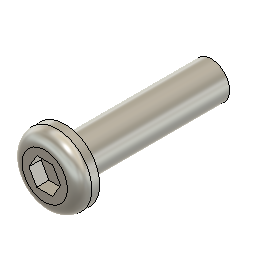
_bolt.35465e34-b387-4346-8fbb-dc58b0572cbc (Autodesk Fusion 360 design; units mm, degrees)
Autodesk Fusion 360 part; units mm, degrees
sketch "Sketch1" plane through (0, 0, 0) normal (0, 0, 1) x (1, 0, 0)
  circle A0 centre (0, 0) radius 2.85
  dimension "d1" = 5.7
  constraint coincident A0.centre origin
  measures "d1" diameter of A0
extrude "Extrude1" add sketch "Sketch1" along normal blind 1.65
fillet "Fillet1" radius 1 1 edges at (-2.6571, -1.0306, 1.65)
sketch "Sketch2" plane through (0, 0, 1.65) normal (0, 0, 1) x (1, 0, 0)
  circle A0 centre (0, 0) radius 1.85
  line L0 (-0.641, 1.131) -> (-1.3, 0.0104)
  line L1 (-1.3, 0.0104) -> (-0.659, -1.1206)
  line L2 (-0.659, -1.1206) -> (0.641, -1.131)
  line L3 (0.641, -1.131) -> (1.3, -0.0104)
  line L4 (1.3, -0.0104) -> (0.659, 1.1206)
  line L5 (0.659, 1.1206) -> (-0.641, 1.131)
  dimension "d6" = 1.3
  constraint coincident A0.centre origin
  measures "d6" distance of L0.start A0.centre
extrude "Extrude2" cut sketch "Sketch2" against normal blind 1 contours L0 L1 L2 L3 L4 L5
sketch "Sketch3" plane through (0, 0, 0) normal (0, 0, -1) x (-1, 0, 0)
  circle A0 centre (0, 0) radius 2.85
  circle A1 centre (0, 0) radius 1.5
  dimension "d9" = 3
  constraint coincident A0.centre A1.centre
  measures "d9" diameter of A1
extrude "Extrude3" add sketch "Sketch3" along normal blind 12 contours A1
